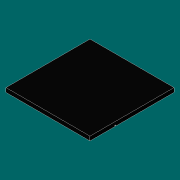
# Autodesk Inventor part: topBottom
Saved by Autodesk Inventor 2016 (Build 200138000, 138)
## iProperties
Created: 2015-10-13
Part Number: topBottom
Material: PC/ABS Plastic
Document SubType Name: Modeling
Designer: Sawaiz
Density: 0.357273 g/cm^3
Appearance: Smooth - Black
Author: Sawaiz
Autodesk Inventor part; units mm, degrees
ref_plane "YZ Plane" through (0, 0, 0) normal (1, 0, 0) x (0, 1, 0)
ref_plane "XZ Plane" through (0, 0, 0) normal (0, 1, 0) x (-1, 0, 0)
ref_plane "XY Plane" through (0, 0, 0) normal (0, 0, 1) x (1, 0, 0)
sketch "Sketch1" plane through (0, 0, 0) normal (0, 0, 1) x (1, 0, 0)
  line L0 (-73.025, -63.5) -> (73.025, -63.5)
  line L1 (73.025, -63.5) -> (73.025, 63.5)
  line L2 (73.025, 63.5) -> (-73.025, 63.5)
  line L3 (-73.025, 63.5) -> (-73.025, -63.5)
  line L4 (-73.025, -63.5) -> (73.025, 63.5) construction
  line L5 (73.025, -63.5) -> (-73.025, 63.5) construction
  point P0 (0, 0)
  dimension "d0" = 146.05
  dimension "d1" = 127
  constraints: 12 end point, 2 midpoint, 2 parallel, 1 horizontal, 1 perpendicular
  measures "d0" distance of L2.end L1.end
  measures "d1" distance of L1.end L0.end
extrude "Extrusion1" add sketch "Sketch1" along normal blind 6.35
sketch "Sketch16" plane through (0, 0, 0) normal (0, 0, -1) x (-1, 0, 0)
  line L0 (-73.025, 63.5) -> (73.025, 63.5) projected
  line L1 (73.025, -63.5) -> (-73.025, -63.5) projected
  line L2 (-35.7188, 63.5) -> (-34.1313, 63.5)
  line L3 (-34.1313, 63.5) -> (-34.1313, -63.5)
  line L4 (-34.1313, -63.5) -> (-35.7187, -63.5)
  line L5 (-35.7187, -63.5) -> (-35.7188, 63.5)
  line L6 (-73.025, -63.5) -> (-73.025, 63.5) projected
  point P0 (0, 0)
  dimension "d114" = 1.5875
  dimension "d115" = 37.3062
  constraints: 8 end point, 2 parallel, 2 point on line, 1 horizontal, 1 perpendicular
  measures "d114" distance between parallel lines of L3 L5
  measures "d115" distance between parallel lines of L6 L5
extrude "Extrusion9" cut sketch "Sketch16" against normal blind 1.5875 contours L0 L3 L1 L5
equation "\"width\" = 127"
equation "\"depth\" = 146.05"
equation "\"plasticThickness\" = 6.35"
equation "\"aerogelHolderDepth\" = 37.30625"
equation "\"height\" = 127"
equation "\"mirrorAngle\" = 5deg"
equation "\"mirrorThickness\" = 3.175"
equation "\"fresnelThickness\" = 0.1"
equation "\"focalLength\" = 76.2"
equation "\"ior\" = 1.49"
equation "\"centerThickness\" = 1.524"
equation "\"fresnelAngle\" = 90deg"
equation "\"fresnelEffectiveDiameter\" = 152.4"
body "Solid1"
